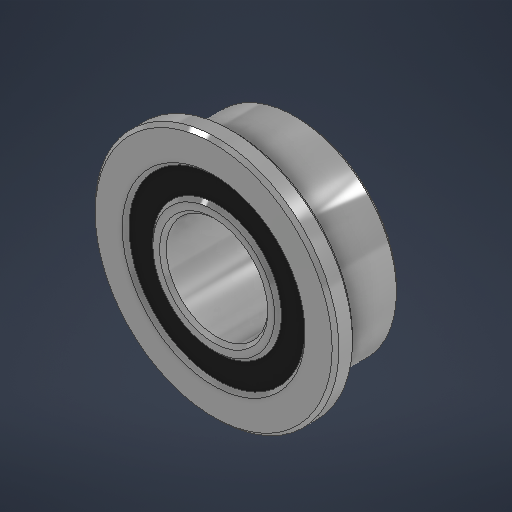
# Autodesk Inventor part: Miniatur Flanschkugellager MF 74 ZZ
Saved by Autodesk Inventor 2026.1 (Build 301233020, 233B)
## iProperties
Created: 2026-04-16
Part Number: Miniatur Flanschkugellager MF 74 ZZ
Material: Generic
Document SubType Name: Modeling
Designer: Bahaa
Mass: 0.0578985 g
Surface Area: 1.3662 cm^2
Volume: 0.0578985 cm^3
Density: 1 g/cm^3
Appearance: Default
Author: Bahaa
Autodesk Inventor part; units mm, degrees
ref_plane "YZ Plane" through (0, 0, 0) normal (1, 0, 0) x (0, 1, 0)
ref_plane "XZ Plane" through (0, 0, 0) normal (0, 1, 0) x (-1, 0, 0)
ref_plane "XY Plane" through (0, 0, 0) normal (0, 0, 1) x (1, 0, 0)
sketch "Sketch1" plane through (0, 0, 0) normal (0, 1, 0) x (-1, 0, 0)
  circle A0 centre (0, 0) radius 3
  circle A1 centre (0, 0) radius 1.5
  circle A2 centre (0, 0) radius 3.6
  circle A3 centre (0, 0) radius 1.9
  circle A4 centre (0, 0) radius 2.6
  dimension "d0" = 6
  dimension "d1" = 3
  dimension "d2" = 7.2
  dimension "d3" = 0.4
  dimension "d4" = 0.4
  constraints: 5 centre point, 3 coincident
  measures "d0" diameter of A0
  measures "d1" diameter of A1
  measures "d2" diameter of A2
  measures "d3" radial gap between concentric circles of A1 A3
  measures "d4" radial gap between concentric circles of A0 A4
extrude "Extrusion1" add sketch "Sketch1" along normal blind 2.5 contours A0 | A3 | A4
extrude "Extrusion2" add sketch "Sketch1" along normal blind 0.6 contours A2
extrude "Extrusion3" cut sketch "Sketch1" along normal blind 0.1 contours A4
extrude "Extrusion4" cut sketch "Sketch1" against normal blind 0.1 from surface at 2.5 contours A4
chamfer "Chamfer1" distance 0.1 angle 45 10 edges at (3, 0.6, 0) (3, 2.5, 0) (2.6, 2.5, 0) (1.9, 2.5, 0) (1.5, 2.5, 0) (3.6, 0.6, 0) (3.6, 0, 0) (2.6, 0, 0) (1.9, 0, 0) (1.5, 0, 0)
body "Solid1"
